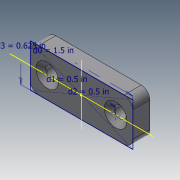
# Autodesk Inventor part: VP PUSHER DETENT
Saved by Autodesk Inventor 2018.3 (Build 223284000, 284)
## iProperties
Created: 2019-11-01
Material: Generic
Vendor: HHMI: JRC - ID&F
Document SubType Name: Modeling
Designer: arnoldj
Density: 1 g/cm^3
Appearance: Default
RuleStatus: InUse
AfterDocSave0: file://Part Number Cleaner
DESIGN DEPARTMENT: HHMI: JRC - ID&F
ALTERED ITEM PART NUMBER: N/A
ALTERED ITEM VENDOR: N/A
ALTERED ITEM DESCRIPTION: N/A
Author: arnoldj
Revision Number: 0
Autodesk Inventor part; units mm, degrees
ref_plane "YZ Plane" through (0, 0, 0) normal (1, 0, 0) x (0, 1, 0)
ref_plane "XZ Plane" through (0, 0, 0) normal (0, 1, 0) x (-1, 0, 0)
ref_plane "XY Plane" through (0, 0, 0) normal (0, 0, 1) x (1, 0, 0)
sketch "Sketch1" plane through (0, 0, 0) normal (0, 0, 1) x (1, 0, 0)
  line L0 (0, 11.1125) -> (0, -11.1125) projected
  line L1 (-26.67, 0) -> (26.67, 0) projected
  line L2 (19.05, -7.9375) -> (-19.05, -7.9375)
  line L3 (-19.05, -7.9375) -> (-19.05, 7.9375)
  line L4 (-19.05, 7.9375) -> (19.05, 7.9375)
  line L5 (19.05, 7.9375) -> (19.05, -7.9375)
  line L6 (19.05, -7.9375) -> (-19.05, 7.9375) construction
  line L7 (-19.05, -7.9375) -> (19.05, 7.9375) construction
  point P0 (0, 0)
  point P1 (-12.7, 0)
  point P2 (12.7, 0)
  dimension "d0" = 38.1
  dimension "d1" = 12.7
  dimension "d2" = 12.7
  dimension "d3" = 15.875
  constraints: 12 end point, 2 midpoint, 2 parallel, 2 point on line, 1 horizontal, 1 perpendicular
  measures "d0" distance of L3.end L4.end
  measures "d1" distance from line of L0 point (-12.7, 0)
  measures "d2" distance from line of L0 point (12.7, 0)
  measures "d3" distance of L2.end L3.end
extrude "Extrusion1" add sketch "Sketch1" against normal blind 6.35
hole "Hole1" at (-12.7, 0, 0) at (12.7, 0, 0) direction (0, 0, -1) diameter 4.4958 end through all countersink diameter 8.4328 countersink angle 100 clearance for "Flat Head Machine Screw (100)" size "#8" standard "Ansi Unified Screw Threads"
fillet "Fillet1" radius 3.175 4 edges at (-19.05, 7.9375, -3.175) (19.05, 7.9375, -3.175) (19.05, -7.9375, -3.175) (-19.05, -7.9375, -3.175)
body "Solid1"
